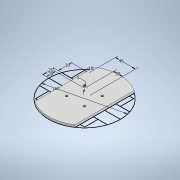
# Autodesk Inventor part: heheheha
Saved by Autodesk Inventor 2020 (Build 240168000, 168)
## iProperties
Created: 2022-12-15
Part Number: heheheha
Material: Ogólny
Document SubType Name: Modeling
Designer: User
Density: 1 g/cm^3
Appearance: Domyślna
Author: User
Autodesk Inventor part; units mm, degrees
ref_plane "YZ Plane" through (0, 0, 0) normal (1, 0, 0) x (0, 1, 0)
ref_plane "XZ Plane" through (0, 0, 0) normal (0, 1, 0) x (-1, 0, 0)
ref_plane "XY Plane" through (0, 0, 0) normal (0, 0, 1) x (1, 0, 0)
sketch "Szkic1" plane through (0, 0, 0) normal (0, 1, 0) x (-1, 0, 0)
  circle A0 centre (0, 0) radius 80
  line L0 (55, -25) -> (45, -25)
  line L1 (45, -25) -> (45, -55)
  line L2 (45, -55) -> (55, -55)
  line L3 (55, -55) -> (55, -25)
  line L4 (55, 25) -> (45, 25)
  line L5 (45, 25) -> (45, 55)
  line L6 (45, 55) -> (55, 55)
  line L7 (55, 55) -> (55, 25)
  line L8 (80, 0) -> (-80, 0)
  line L9 (0, 80) -> (0, -80)
  line L10 (-45, -25) -> (-55, -25)
  line L11 (-55, -25) -> (-55, -55)
  line L12 (-55, -55) -> (-45, -55)
  line L13 (-45, -55) -> (-45, -25)
  line L14 (-45, 55) -> (-55, 55)
  line L15 (-55, 55) -> (-55, 25)
  line L16 (-55, 25) -> (-45, 25)
  line L17 (-45, 25) -> (-45, 55)
  circle A1 centre (20, -20) radius 2.5
  circle A2 centre (20, 20) radius 2.5
  circle A3 centre (-20, -20) radius 2.5
  circle A4 centre (-20, 20) radius 2.5
  line L18 (45, -55) -> (45, -66.1438)
  line L19 (55, -25) -> (75.9934, -25)
  line L20 (45, 55) -> (45, 66.1438)
  line L21 (55, 25) -> (75.9934, 25)
  line L22 (-45, -55) -> (-45, -66.1438)
  line L23 (-55, -25) -> (-75.9934, -25)
  line L24 (-55, 25) -> (-75.9934, 25)
  line L25 (-45, 55) -> (-45, 66.1438)
  line L26 (45, -25) -> (45, 25)
  line L27 (-45, -25) -> (-45, 25)
  dimension "d0" = 160
  dimension "d1" = 10
  dimension "d2" = 30
  dimension "d3" = 25
  dimension "d4" = 45
  dimension "d5" = 5
  dimension "d6" = 20
  dimension "d7" = 20
  constraints: 56 end point, 9 symmetric about line, 8 parallel, 6 perpendicular, 6 point on circle, 5 centre point, 5 horizontal, 2 midpoint, 1 coincident, 1 collinear, 1 vertical, 16 other
  measures "d0" diameter of A0
  measures "d1" distance of L1.end L2.end
  measures "d2" distance of L2.end L0.start
  measures "d3" distance between parallel lines of L0 L8
  measures "d4" distance between parallel lines of L1 L9
  measures "d5" diameter of A1
  measures "d6" distance from line of L9 A1.centre
  measures "d7" distance from line of L8 A1.centre
extrude "Wyciągnięcie proste1" add sketch "Szkic1" along normal blind 5 contours L26 L1 L18 A0 L9 L8 | L8 L9 A0 L20 L5 L26 | L9 A0 L22 L13 L27 L8 | L8 L27 L17 L25 A0 L9
extrude "Wyciągnięcie proste2" add sketch "Szkic1" along normal blind 2.5 contours A1 | A2 | A3 | A4
hole "Otwór1" at (-20, 0, 20) at (20, 0, 20) at (20, 0, -20) at (-20, 0, -20) direction (0, 1, 0) diameter 2 depth 2.5
fillet "Zaokrąglenie1" radius 2 1 edges at (0, 0, -80)
